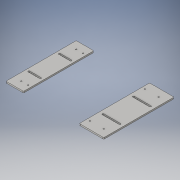
# Autodesk Inventor part: vrRig_v08_slideMountBottom
Saved by Autodesk Inventor 2016 (Build 200138000, 138)
## iProperties
Created: 2018-03-28
Part Number: vrRig_v08_slideMountBottom
Material: Generic
Document SubType Name: Modeling
Designer: harveylab
Density: 1 g/cm^3
Appearance: Default
Author: harveylab
Autodesk Inventor part; units mm, degrees
ref_plane "YZ Plane" through (0, 0, 0) normal (1, 0, 0) x (0, 1, 0)
ref_plane "XZ Plane" through (0, 0, 0) normal (0, 1, 0) x (-1, 0, 0)
ref_plane "XY Plane" through (0, 0, 0) normal (0, 0, 1) x (1, 0, 0)
sketch "Sketch1" plane through (0, 0, 0) normal (0, 1, 0) x (-1, 0, 0)
  line L0 (0, 0) -> (304.8, 0) construction
  line L1 (304.8, 0) -> (304.8, -304.8) construction
  line L2 (304.8, -304.8) -> (0, -304.8) construction
  line L3 (0, -152.4) -> (304.8, -152.4) construction
  line L4 (31.75, -38.1) -> (88.9, -38.1) construction
  line L5 (88.9, -38.1) -> (346.202, -38.1) construction
  line L6 (346.202, -38.1) -> (374.65, -38.1) construction
  line L7 (374.65, -38.1) -> (406.4, -38.1) construction
  circle A0 centre (31.75, -38.1) radius 2.54
  circle A1 centre (88.9, -38.1) radius 2.54
  circle A2 centre (346.202, -38.1) radius 2.54
  circle A3 centre (374.65, -38.1) radius 2.54
  line L8 (101.6, -9.525) -> (101.6, -152.4)
  circle A4 centre (31.75, -266.7) radius 2.54
  circle A5 centre (88.9, -266.7) radius 2.54
  line L9 (101.6, -295.275) -> (101.6, -152.4)
  line L10 (88.9, -88.9) -> (88.9, -88.9)
  line L11 (85.725, -85.725) -> (15.875, -85.725)
  line L12 (12.7, -88.9) -> (12.7, -89.154)
  line L13 (15.875, -92.329) -> (85.725, -92.329)
  arc A6 (88.9, -88.9) -> (85.725, -85.725) centre (85.725, -88.9) ccw
  arc A7 (85.725, -92.329) -> (88.9, -89.154) centre (85.725, -89.154) ccw
  arc A8 (15.875, -85.725) -> (12.7, -88.9) centre (15.875, -88.9) ccw
  arc A9 (12.7, -89.154) -> (15.875, -92.329) centre (15.875, -89.154) ccw
  line L14 (88.9, -88.9) -> (88.9, -89.154)
  line L15 (88.9, -215.9) -> (88.9, -215.9)
  line L16 (85.725, -219.075) -> (15.875, -219.075)
  line L17 (12.7, -215.9) -> (12.7, -215.646)
  line L18 (15.875, -212.471) -> (85.725, -212.471)
  arc A10 (85.725, -219.075) -> (88.9, -215.9) centre (85.725, -215.9) ccw
  arc A11 (88.9, -215.646) -> (85.725, -212.471) centre (85.725, -215.646) ccw
  arc A12 (12.7, -215.9) -> (15.875, -219.075) centre (15.875, -215.9) ccw
  arc A13 (15.875, -212.471) -> (12.7, -215.646) centre (15.875, -215.646) ccw
  line L19 (88.9, -215.9) -> (88.9, -215.646)
  arc A14 (98.425, -298.45) -> (101.6, -295.275) centre (98.425, -295.275) ccw
  arc A15 (101.6, -9.525) -> (98.425, -6.35) centre (98.425, -9.525) ccw
  line L20 (346.202, -38.1) -> (333.502, -38.1) construction
  line L21 (333.502, -38.1) -> (333.502, -9.525)
  line L22 (406.4, -69.85) -> (406.4, -152.4)
  line L23 (333.502, -38.1) -> (333.502, -152.4)
  circle A16 centre (393.7, -88.9) radius 3.302
  line L24 (393.7, -85.598) -> (346.202, -85.598)
  line L25 (346.202, -85.598) -> (346.202, -92.202)
  line L26 (346.202, -92.202) -> (393.7, -92.202)
  line L27 (393.7, -92.202) -> (393.7, -85.598)
  circle A17 centre (346.202, -88.9) radius 3.302
  line L28 (88.9, -266.7) -> (346.202, -266.7) construction
  line L29 (346.202, -266.7) -> (374.65, -266.7) construction
  line L30 (374.65, -266.7) -> (406.4, -266.7) construction
  circle A18 centre (346.202, -266.7) radius 2.54
  circle A19 centre (374.65, -266.7) radius 2.54
  line L31 (346.202, -266.7) -> (333.502, -266.7) construction
  line L32 (333.502, -266.7) -> (333.502, -295.275)
  line L33 (406.4, -234.95) -> (406.4, -152.4)
  line L34 (333.502, -266.7) -> (333.502, -152.4)
  circle A20 centre (393.7, -215.9) radius 3.302
  line L35 (393.7, -219.202) -> (346.202, -219.202)
  line L36 (346.202, -219.202) -> (346.202, -212.598)
  line L37 (346.202, -212.598) -> (393.7, -212.598)
  line L38 (393.7, -212.598) -> (393.7, -219.202)
  circle A21 centre (346.202, -215.9) radius 3.302
  line L39 (98.425, -298.45) -> (3.175, -298.45)
  line L40 (0, -295.275) -> (0, -9.525)
  line L41 (3.175, -6.35) -> (98.425, -6.35)
  line L42 (406.4, -234.95) -> (406.4, -295.275)
  line L43 (403.225, -298.45) -> (336.677, -298.45)
  line L44 (336.677, -6.35) -> (403.225, -6.35)
  line L45 (406.4, -9.525) -> (406.4, -69.85)
  arc A22 (3.175, -6.35) -> (0, -9.525) centre (3.175, -9.525) ccw
  arc A23 (0, -295.275) -> (3.175, -298.45) centre (3.175, -295.275) ccw
  arc A24 (403.225, -298.45) -> (406.4, -295.275) centre (403.225, -295.275) ccw
  arc A25 (333.502, -295.275) -> (336.677, -298.45) centre (336.677, -295.275) ccw
  arc A26 (406.4, -9.525) -> (403.225, -6.35) centre (403.225, -9.525) ccw
  arc A27 (336.677, -6.35) -> (333.502, -9.525) centre (336.677, -9.525) ccw
  line L46 (98.425, -298.45) -> (3.175, -298.45)
  line L47 (0, -295.275) -> (0, -9.525)
  line L48 (3.175, -6.35) -> (98.425, -6.35)
  line L49 (101.6, -9.525) -> (101.6, -295.275)
  arc A28 (98.425, -298.45) -> (101.6, -295.275) centre (98.425, -295.275) ccw
  arc A29 (0, -295.275) -> (3.175, -298.45) centre (3.175, -295.275) ccw
  arc A30 (3.175, -6.35) -> (0, -9.525) centre (3.175, -9.525) ccw
  arc A31 (101.6, -9.525) -> (98.425, -6.35) centre (98.425, -9.525) ccw
  point P0 (101.6, -6.35)
  point P1 (101.6, -298.45)
  point P2 (12.7, -92.329)
  point P3 (12.7, -85.725)
  point P4 (12.7, -212.471)
  point P5 (12.7, -219.075)
  point P6 (333.502, -6.35)
  point P7 (333.502, -298.45)
  point P8 (406.4, -6.35)
  dimension "d53" = 6.604
  dimension "d0" = 304.8
  dimension "d1" = 304.8
  dimension "d6" = 57.15
  dimension "d7" = 257.302
  dimension "d8" = 28.448
  dimension "d9" = 31.75
  dimension "d10" = 5.08
  dimension "d11" = 5.08
  dimension "d12" = 5.08
  dimension "d13" = 5.08
  dimension "d41" = 6.604
  dimension "d42" = 3.175
  dimension "d44" = 12.7
  dimension "d45" = 31.75
  dimension "d58" = 3.175
  dimension "d59" = 3.175
  constraints: 100 end point, 40 point on circle, 33 symmetric about line, 29 tangent, 28 centre point, 22 point on line, 11 equal radius, 10 horizontal, 9 perpendicular, 7 parallel, 6 coincident, 5 vertical, 4 vertical alignment, 1 midpoint, 16 other
  measures "d0" distance of L1.end L2.end
  measures "d1" distance of L0.end L1.end
  measures "d6" distance of L4.start L4.end
  measures "d7" distance of L4.end L5.end
  measures "d8" distance of L5.end L6.end
  measures "d9" distance of L6.end L7.end
  measures "d10" diameter of A0
  measures "d11" diameter of A1
  measures "d12" diameter of A2
  measures "d13" diameter of A3
  measures "d41" distance of point (12.7, -92.329) point (12.7, -85.725)
  measures "d42" radius of A6
  measures "d44" distance of L20.start L20.end
  measures "d45" distance of L20.end point (333.502, -6.35)
  measures "d58" radius of A22
  measures "d59" radius of A28
extrude "Extrusion2" add sketch "Sketch1" along normal blind 6.35
body "Solid2"
